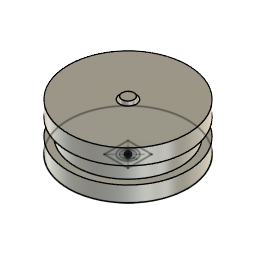
U_Wheel v2 (Autodesk Fusion 360 design; units mm, degrees)
Autodesk Fusion 360 part; units mm, degrees
sketch "Sketch1" plane through (0, 0, 0) normal (0, 0, 1) x (1, 0, 0)
  circle A0 centre (0, 0) radius 25
  circle A1 centre (0, 0) radius 3.5
  line L0 (5, -5) -> (-5, -5)
  line L1 (-5, -5) -> (-5, 5)
  line L2 (-5, 5) -> (5, 5)
  line L3 (5, 5) -> (5, -5)
  line L4 (5, -5) -> (-5, 5) construction
  line L5 (-5, -5) -> (5, 5) construction
  circle A2 centre (0, 0) radius 2.5
  dimension "d1" = 50
  dimension "d13" = 7
  dimension "d17" = 10
  dimension "d18" = 10
  dimension "d26" = 5
  constraint coincident A0.centre A1.centre
  constraint concentric A0 A1
  constraint horizontal L0
  constraint perpendicular L0 L1
  constraint parallel L0 L2
  constraint parallel L1 L3
  constraint coincident L4 A0.centre
  constraint coincident L5 A0.centre
  constraint concentric A1 A2
  measures "d1" diameter of A0
  measures "d13" diameter of A1
  measures "d17" distance of L1.end L2.end
  measures "d18" distance of L0.end L1.end
  measures "d26" diameter of A2
extrude "Extrude1" add sketch "Sketch1" along normal blind 20 contours A0 | A1 | L0 L1 L2 L3 | A2 makes body 1
sketch "Sketch6" plane through (0, 0, 0) normal (1, 0, 0) x (0, 1, 0)
  line L0 (0, 20) -> (-25, 20)
  line L1 (25, 20) -> (0, 20)
  line L2 (0, 0) -> (-25, 0)
  line L3 (25, 0) -> (0, 0)
  line L4 (25, 0) -> (25, 20)
  line L5 (-25, 0) -> (-25, 20)
  line L6 (-25, 13.5) -> (-22, 13.5)
  line L7 (-22, 13.5) -> (-22, 6.5)
  line L8 (-22, 6.5) -> (-25, 6.5)
  line L9 (-25, 6.5) -> (-25, 13.5)
  dimension "d7" = 3
  dimension "d8" = 7
  dimension "d9" = 6.5
  constraint horizontal L6
  constraint vertical L7
  constraint horizontal L8
  constraint vertical L9
  constraint coincident L5 L6.start
  measures "d7" distance of L6.start L6.end
  measures "d8" distance of L6.start L8.end
  measures "d9" distance of L0 L6
revolve "Revolve1" cut sketch "Sketch6" angle 360 about axis through (0, 0, 0) along (0, 0, -1) contours L5 L6 L7 L8 L9 bodies 1
extrude "Extrude2" cut sketch "Sketch1" along normal blind 24.171 contours A1 | A2 bodies 1
extrude "Extrude5" add sketch "Sketch1" along normal blind 20.071 separate body contours A2 makes body 2
extrude "Extrude3" add sketch "Sketch1" along normal blind 1.5137 contours L0 L1 L2 L3 bodies 1
ref_plane "WorkPlane1" through (30, 0, 0) normal (1, 0, 0) x (0, 1, 0)
extrude "Extrude6" add sketch "Sketch1" against normal blind 1.9941 contours A2 bodies 2
extrude "Extrude7" add 1 faces at (-0.7508, 0.3616, 20.071) along direction (0, 0, 1) blind 1.078 on bodies 2 bodies 2
equation "d1 = rope_wheel"
equation "rope_wheel = 50 mm"
equation "rope_wheel_hohe = 20 mm"
equation "rope_u_kanal = 10 mm"
equation "d5 = rope_wheel_hohe"
equation "rope_wheel_D_klein = 7 mm"
equation "d13 = rope_wheel_D_klein"
equation "rope_stützt_arm_lange = 10 mm"
equation "d17 = rope_stützt_arm_lange"
equation "d18 = rope_stützt_arm_lange"
